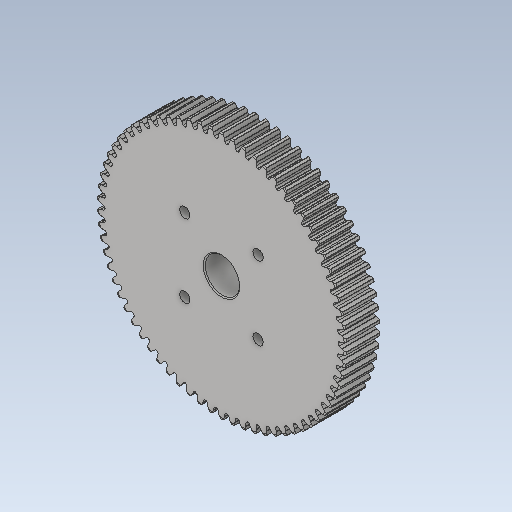
# Autodesk Inventor part: GEABP1.0-70-10-B-10-KFC30-K3_b
Saved by Autodesk Inventor 2020.2 (Build 242310000, 310)
## iProperties
Created: 2022-11-02
Part Number: GEABP1.0-70-10-B-10-KFC30-K3_b
Material: Generic
Catalog Web Link: www.cadenas.de
Description: GEABM, GEABMS, GEABMT, GEABP, GEABPS, GEABPT, GEABA, GEABAS, GEABAT_body-Plastic Spur Gears - Pressure Angle 20 Degrees, Module 0.5/0.8/1.0/1.5/2.0/2.5/3.0
Vendor: MISUMI
Document SubType Name: Modeling
Designer: psAdmin
Manufacturer: MISUMI
Mass: 48.5724 g
Surface Area: 144.734 cm^2
Volume: 48.5724 cm^3
Density: 1 g/cm^3
Appearance: PSOLRGB-175-175-175
Category: PARTsolutions
Company: MISUMI
PSOL_IDENT_0: {$CADENAS_DATA/23d-libs/misumi/metric/54_spur_gears/geabms20/geabms20.prj},408 {VTYP=3D},{NB=GEABP1.
PSOL_IDENT_1: 0-70-10-B-10-KFC30-K3_b},{LINA=GEABP1.0-70-10-B-10-KFC30-K3},{NN=GEABM, GEABMS, GEABMT, GEABP, GEABP
PSOL_IDENT_2: S, GEABPT, GEABA, GEABAS, GEABAT_body},{DATE=17.10.2022 23:48:33},{GEOMDATE=14.09.2022 05:11:00},{VE
PSOL_IDENT_3: RSION=},{LINEID=30},{WBVAR=MATSG,MATCR,NT,B,TS,PS,ALT1,ALT2,TPC,ALT11,ALT10,BS,ALT3,Z,J,ALT4,Q,R,S,T
PSOL_IDENT_4: ,ALT5,LFC,LTC,MALT5,ALT6,KFC,KTC,K},{WBNUMERIC=NT,B,BS,Z,J,Q,R,S,T,LFC,LTC,KFC,KTC,K}  {NB=GEABP1.0-
PSOL_IDENT_5: 70-10-B-10-KFC30-K3_b},{LINA=GEABP1.0-70-10-B-10-KFC30-K3},{KT=DUMMY},{PN=GEABP1.0-70-10-B-10-KFC30-
PSOL_IDENT_6: K3},{TYPE=GEABP},{MATSG=PW},{MATSGALG='MCN','MC Nylon','PW','Polyacetal White','PB','Polyacetal Blue'
PSOL_IDENT_7: },{MATCR=},{MATCRALG='','-','S45C','1045 Carbon Steel','SUS304','304 Stainless Steel'},{MOD=1.0},{MO
PSOL_IDENT_8: D1=1.0},{NT=70},{NTALG=15,16,18,20,22,24,25,26,28,30,32,35,36,40,45,48,50,55,60,70,75,80,90,100,120}
PSOL_IDENT_9: ,{B=10},{BALG=10,15},{TS=B},{TSALG='A','A','B','B'},{TSPN=-B},{PS=10},{PSALG='10','10','11','11','12'
PSOL_IDENT_10: ,'12','13','13','14','14','15','15','16','16','17','17','18','18','19','19','20','20','21','21','22'
PSOL_IDENT_11: ,'22','23','23','24','24','25','25','26','26','27','27','28','28'},{PSCRL='10','10','11','11','12','
PSOL_IDENT_12: 12','13','13','14','14','15','15','16','16','17','17','18','18','19','19','20','20','21','21','22','
PSOL_IDENT_13: 22','23','23','24','24','25','25','26','26','27','27','28','28'},{PSCRW='10','10','12','12','15','15'
PSOL_IDENT_14: ,'20','20'},{DD=70.0},{DD05=35},{DD08=56},{DD10=70},{DD15=105},{DD20=0},{DD25=0},{DD30=0},{D=72.0},{
PSOL_IDENT_15: D05=36},{D08=57.6},{D10=72},{D15=108},{D20=0},{D25=0},{D30=0},{G=67.50},{G05=33.75},{G08=54},{G10=67
PSOL_IDENT_16: .5},{G15=101.25},{G20=0},{G25=0},{G30=0},{H=40.0},{L=20},{LL1=10},{LL2=4.0},{M=M4},{M3D=4},{P=10.00}
PSOL_IDENT_17: ,{DD1=0},{CIFR=15},{CIFM=4},{CIFK=0},{CIFTAP=1},{ALT1=},{ALT1ALG='','w/o Set Screw','KC90','with KC9
PSOL_IDENT_18: 0 (Set Screw)','KC120','with KC120 (Set Screw)'},{ALT1PN=},{ALT2=},{ALT2ALG='','w/o TPC (Tapped Hole
PSOL_IDENT_19: Dimension)','TPC','with TPC (Tapped Hole Dimension)'},{TPC=N/A},{TPCALG='N/A'},{ALT2PN=},{KC=0},{AL
PSOL_IDENT_20: T11=},{ALT11ALG='', 'w/o GBA (Gear bottom adjustment of phase focus)', 'GBA', 'with GBA (Gear bottom
PSOL_IDENT_21: adjustment of phase focus)' },{ALT11PN=},{DEG=0},{ALT10=},{ALT10ALG= '','w/o BS (Boss Cut)','BS','w
PSOL_IDENT_22: ith BS (Boss Cut)' },{ALT10PN=},{BS=0.0},{BSALG=0},{BSMIN=7},{BSMINALG=7.000},{BSMAX=10},{LL13D=10},
PSOL_IDENT_23: {LL23D=16},{LBS=20},{ALT3=},{ALT3ALG= '','w/o Stepped Hole','DHL','with DHL (Stepped Hole)','DHR','w
PSOL_IDENT_24: ith DHR (Stepped Hole)' },{ALT3PN=},{ZJPN=},{ALT31=1},{ALT32=1},{Z=0},{ZALG=0},{ZMINL=12},{ZMAXL=63}
PSOL_IDENT_25: ,{ZMINR=12},{ZMAXR=36},{ZPN=},{J=0.0},{JALG=0},{JMIN=2},{JMAX=0},{JPN=},{ALT4=},{ALT4ALG= '','w/o WD
PSOL_IDENT_26: H (Both Ends Stepped Hole)','WDH','with WDH (Both Ends Stepped Hole)' },{ALT4PN=},{QRSTPN=},{LB=20.0
PSOL_IDENT_27: 00},{Q=0},{QALG=0},{QMIN=12},{QMAX=36},{QPN=},{R=0},{RALG=0},{RMIN=12},{RMAX=36},{RPN=},{S=0},{SALG=
PSOL_IDENT_28: 0},{SMIN=3},{SMAX=14},{SPN=},{T=0},{TALG=0},{TMIN=3},{TMAX=0},{TPN=},{ALT5=},{ALT5ALG= '','Not appli
PSOL_IDENT_29: cable' },{LFC=0},{LFCALG=0},{LTC=0},{LTCALG=0},{LPCDMIN=18},{LPCDMAX=60},{LCMAX=63},{MALT5=N/A},{MAL
PSOL_IDENT_30: T5ALG= 'N/A' },{LCMAX2=60},{C=0.0},{ALT5PN=},{ALT6=KFC},{ALT6ALG= '','w/o Side Through Hole','KFC','
PSOL_IDENT_31: with KFC (Side Through Hole)','KTC','with KTC (Side Through Hole)' },{ALT6PN=-KFC},{KFTCPN=30-K3},{K
PSOL_IDENT_32: FC=30},{KFCALG=[17:33/1],[47:60/1]},{KFCPN=30},{KTC=0},{KTCALG=[0]},{KTCPN=},{KPCDMIN1=17},{KPCDMAX1=
PSOL_IDENT_33: 33},{KPCDMIN2=47},{KPCDMAX2=60},{K=3.0},{KALG=[3:6/0.5]},{KPCD=30},{KPN=-K3},{SCREW=4},{SCREWL=3},{A
PSOL_IDENT_34: G=0},{PCD=30},{SHN=4},{SHDEG1=45},{SHDEG2=90},{PZQRDD2=10},{D1=1.285714},{D2=2.571429},{D3=20},{D4=0
PSOL_IDENT_35: .1},{D5=11.666667},{D6=10.769231},{D7=0.85},{D8=0.5},{D9=0.82917},{S1=15},{S2=0.5},{KR=15}
NB: GEABP1.0-70-10-B-10-KFC30-K3_b
NN: GEABM, GEABMS, GEABMT, GEABP, GEABPS, GEABPT, GEABA, GEABAS, GEABAT_body
NT: 70
NBSYN: $PN._b
LINA: GEABP1.0-70-10-B-10-KFC30-K3
CATALOG: Misumi
PN: GEABP1.0-70-10-B-10-KFC30-K3
MATSG: Polyacetal White
MATCR: -
MOD: 1.0
B: 10
TS: B
PS: 10
DD: 70
D: 72
G: 67.5
H: 40
L: 20
LL1: 10
LL2: 4
M: M4
DD1: 0
ALT1: w/o Set Screw
ALT2: w/o TPC (Tapped Hole Dimension)
TPC: N/A
ALT11: w/o GBA (Gear bottom adjustment of phase focus)
ALT10: w/o BS (Boss Cut)
BS: 0
ALT3: w/o Stepped Hole
Z: 0
J: 0
ALT4: w/o WDH (Both Ends Stepped Hole)
Q: 0
R: 0
S: 0
T: 0
ALT5: Not applicable
LFC: 0
LTC: 0
MALT5: N/A
C: 0
ALT6: with KFC (Side Through Hole)
KFC: 30
KTC: 0
K: 3
SUPPLIER: MISUMI
ARTICLENO: GEABP1.0-70-10-B-10-KFC30-K3_b
BOMINFO: GEABP1.0-70-10-B-10-KFC30-K3
CREATOR: CADENAS GmbH
Title: GEABP1.0-70-10-B-10-KFC30-K3
Author: Cadenas PARTsolutions
Comments: Plastic Spur Gears - Pressure Angle 20 Degrees, Module 0.5/0.8/1.0/1.5/2.0/2.5/3.0
Autodesk Inventor part; units mm, degrees
(part 1 of 2)
sketch "Sketch_2" plane through (0, 0, 0) normal (1, 0, 0) x (0, 1, 0)
  line L0 (0, -500) -> (0, 500)
  line L1 (0, 0) -> (35.5, 0)
  line L2 (35.5, 0) -> (38, -0.6699)
  line L3 (38, -0.6699) -> (38, -9.3301)
  line L4 (38, -9.3301) -> (35.5, -10)
  line L5 (35.5, -10) -> (20, -10)
  line L6 (20, -10) -> (20, -19.7)
  line L7 (20, -19.7) -> (19.7, -20)
  line L8 (19.7, -20) -> (0, -20)
  line L9 (0, -20) -> (0, 0)
  constraints: 20 end point
revolve "Revolution1" add sketch "Sketch_2" angle 360 about axis through (0, 0, -500) along (0, 0, -1)
sketch "_____12" plane through (0, 0, 0) normal (0, 0, 1) x (1, 0, 0)
  circle A0 centre (0, 0) radius 144
  arc A1 (-35.9769, 1.2884) -> (-35.9213, 1.1952) centre (-35.877, 1.2849) ccw
  arc A2 (-35.9213, 1.1952) -> (-34.9912, 0.7853) centre (-30.756, 11.6561) ccw
  arc A3 (-34.9912, 0.7853) -> (-34.8755, 0.7497) centre (-34.6902, 1.5579) ccw
  arc A4 (-34.1021, 0.5416) -> (-34.8755, 0.7497) centre (-37.2859, -9.7463) ccw
  arc A5 (-33.7499, 0.063) -> (-34.1021, 0.5416) centre (-34.2499, 0.0639) ccw
  arc A6 (-33.7499, 0.063) -> (-33.7499, -0.063) centre (0, 0) ccw
  arc A7 (-34.1021, -0.5416) -> (-33.7499, -0.063) centre (-34.2499, -0.0639) ccw
  arc A8 (-34.8755, -0.7497) -> (-34.1021, -0.5416) centre (-37.2859, 9.7463) ccw
  arc A9 (-34.8755, -0.7497) -> (-34.9912, -0.7853) centre (-34.6902, -1.5579) ccw
  arc A10 (-34.9912, -0.7853) -> (-35.9213, -1.1952) centre (-30.756, -11.6561) ccw
  arc A11 (-35.9213, -1.1952) -> (-35.9769, -1.2884) centre (-35.877, -1.2849) ccw
  arc A12 (-35.9769, -1.2884) -> (-35.9476, -1.9417) centre (0, 0) ccw
  arc A13 (-35.9476, -1.9417) -> (-35.8838, -2.0296) centre (-35.8477, -1.9363) ccw
  arc A14 (-35.8838, -2.0296) -> (-34.9207, -2.3544) centre (-31.677, 8.8523) ccw
  arc A15 (-34.9207, -2.3544) -> (-34.8023, -2.3795) centre (-34.6902, -1.5579) ccw
  arc A16 (-34.0134, -2.5175) -> (-34.8023, -2.3795) centre (-36.2622, -13.0493) ccw
  arc A17 (-33.6197, -2.9626) -> (-34.0134, -2.5175) centre (-34.1178, -3.0065) ccw
  arc A18 (-33.6197, -2.9626) -> (-33.6084, -3.0881) centre (0, 0) ccw
  arc A19 (-33.9163, -3.5963) -> (-33.6084, -3.0881) centre (-34.1063, -3.1338) ccw
  arc A20 (-34.6679, -3.8729) -> (-33.9163, -3.5963) centre (-38.0095, 6.3647) ccw
  arc A21 (-34.6679, -3.8729) -> (-34.7799, -3.9188) centre (-34.4109, -4.6613) ccw
  arc A22 (-34.7799, -3.9188) -> (-35.6695, -4.4104) centre (-29.5873, -14.3661) ccw
  arc A23 (-35.6695, -4.4104) -> (-35.7166, -4.5082) centre (-35.6174, -4.4957) ccw
  arc A24 (-35.7166, -4.5082) -> (-35.6288, -5.1562) centre (0, 0) ccw
  arc A25 (-35.6288, -5.1562) -> (-35.5574, -5.238) centre (-35.5299, -5.1419) ccw
  arc A26 (-35.5574, -5.238) -> (-34.5691, -5.4752) centre (-32.343, 5.9771) ccw
  arc A27 (-34.5691, -5.4752) -> (-34.4489, -5.4896) centre (-34.4109, -4.6613) ccw
  arc A28 (-33.6508, -5.5563) -> (-34.4489, -5.4896) centre (-34.9465, -16.2473) ccw
  arc A29 (-33.2188, -5.9643) -> (-33.6508, -5.5563) centre (-33.7109, -6.0527) ccw
  arc A30 (-33.2188, -5.9643) -> (-33.1963, -6.0883) centre (0, 0) ccw
  arc A31 (-33.4574, -6.622) -> (-33.1963, -6.0883) centre (-33.6881, -6.1785) ccw
  arc A32 (-34.1812, -6.965) -> (-33.4574, -6.622) centre (-38.427, 2.932) ccw
  arc A33 (-34.1812, -6.965) -> (-34.2886, -7.0206) centre (-33.8545, -7.7271) ccw
  arc A34 (-34.2886, -7.0206) -> (-35.1306, -7.59) centre (-28.1804, -16.9605) ccw
  arc A35 (-35.1306, -7.59) -> (-35.1687, -7.6917) centre (-35.071, -7.6703) ccw
  arc A36 (-35.1687, -7.6917) -> (-35.0232, -8.3292) centre (0, 0) ccw
  arc A37 (-35.0232, -8.3292) -> (-34.9447, -8.4042) centre (-34.9259, -8.306) ccw
  arc A38 (-34.9447, -8.4042) -> (-33.9391, -8.5519) centre (-32.7486, 3.0538) ccw
  arc A39 (-33.9391, -8.5519) -> (-33.8182, -8.5554) centre (-33.8545, -7.7271) ccw
  arc A40 (-33.0173, -8.5504) -> (-33.8182, -8.5554) centre (-33.3494, -19.3145) ccw
  arc A41 (-32.5504, -8.918) -> (-33.0173, -8.5504) centre (-33.0327, -9.0501) ccw
  arc A42 (-32.5504, -8.918) -> (-32.5169, -9.0395) centre (0, 0) ccw
  arc A43 (-32.7291, -9.5945) -> (-32.5169, -9.0395) centre (-32.9987, -9.1734) ccw
  arc A44 (-33.4192, -10.0009) -> (-32.7291, -9.5945) centre (-38.5351, -0.5244) ccw
  arc A45 (-33.4192, -10.0009) -> (-33.5213, -10.066) centre (-33.0256, -10.7307) ccw
  arc A46 (-33.5213, -10.066) -> (-34.3088, -10.7085) centre (-26.5467, -19.4183) ccw
  arc A47 (-34.3088, -10.7085) -> (-34.3377, -10.8132) centre (-34.2423, -10.7832) ccw
  arc A48 (-34.3377, -10.8132) -> (-34.1356, -11.4351) centre (0, 0) ccw
  arc A49 (-34.1356, -11.4351) -> (-34.0507, -11.5028) centre (-34.0408, -11.4033) ccw
  arc A50 (-34.0507, -11.5028) -> (-33.0359, -11.5598) centre (-32.8905, 0.106) ccw
  arc A51 (-33.0359, -11.5598) -> (-32.9151, -11.5524) centre (-33.0256, -10.7307) ccw
  arc A52 (-32.1179, -11.4756) -> (-32.9151, -11.5524) centre (-31.4838, -22.2261) ccw
  arc A53 (-31.62, -11.7999) -> (-32.1179, -11.4756) centre (-32.0885, -11.9747) ccw
  arc A54 (-31.62, -11.7999) -> (-31.5757, -11.9179) centre (0, 0) ccw
  arc A55 (-31.7373, -12.4897) -> (-31.5757, -11.9179) centre (-32.0435, -12.0944) ccw
  arc A56 (-32.3882, -12.9563) -> (-31.7373, -12.4897) centre (-38.333, -3.9765) ccw
  arc A57 (-32.3882, -12.9563) -> (-32.484, -13.0303) centre (-31.9307, -13.6479) ccw
  arc A58 (-32.484, -13.0303) -> (-33.2108, -13.7408) centre (-24.6991, -21.7197) ccw
  arc A59 (-33.2108, -13.7408) -> (-33.2301, -13.8477) centre (-33.1378, -13.8092) ccw
  arc A60 (-33.2301, -13.8477) -> (-32.9731, -14.449) centre (0, 0) ccw
  arc A61 (-32.9731, -14.449) -> (-32.8825, -14.5088) centre (-32.8815, -14.4088) ccw
  arc A62 (-32.8825, -14.5088) -> (-31.8667, -14.4745) centre (-32.7676, -2.8427) ccw
  arc A63 (-31.8667, -14.4745) -> (-31.747, -14.4564) centre (-31.9307, -13.6479) ccw
  arc A64 (-30.9599, -14.3084) -> (-31.747, -14.4564) centre (-29.3647, -24.9588) ccw
  arc A65 (-30.435, -14.5868) -> (-30.9599, -14.3084) centre (-30.8859, -14.8029) ccw
  arc A66 (-30.435, -14.5868) -> (-30.3803, -14.7003) centre (0, 0) ccw
  arc A67 (-30.49, -15.2843) -> (-30.3803, -14.7003) centre (-30.8304, -14.9181) ccw
  arc A68 (-31.0964, -15.8074) -> (-30.49, -15.2843) centre (-37.8222, -7.3967) ccw
  arc A69 (-31.0964, -15.8074) -> (-31.1852, -15.8897) centre (-30.5788, -16.4552) ccw
  arc A70 (-31.1852, -15.8897) -> (-31.8454, -16.6625) centre (-22.6528, -23.8463) ccw
  arc A71 (-31.8454, -16.6625) -> (-31.8551, -16.7707) centre (-31.7666, -16.7241) ccw
  arc A72 (-31.8551, -16.7707) -> (-31.5452, -17.3465) centre (0, 0) ccw
  arc A73 (-31.5452, -17.3465) -> (-31.4496, -17.398) centre (-31.4576, -17.2983) ccw
  arc A74 (-31.4496, -17.398) -> (-30.4409, -17.2728) centre (-32.3808, -5.7685) ccw
  arc A75 (-30.4409, -17.2728) -> (-30.3234, -17.244) centre (-30.5788, -16.4552) ccw
  arc A76 (-29.5527, -17.026) -> (-30.3234, -17.244) centre (-27.0092, -27.4906) ccw
  arc A77 (-29.0049, -17.2562) -> (-29.5527, -17.026) centre (-29.4346, -17.5119) ccw
  arc A78 (-29.0049, -17.2562) -> (-28.9403, -17.3644) centre (0, 0) ccw
  arc A79 (-28.9971, -17.9559) -> (-28.9403, -17.3644) centre (-29.369, -17.6216) ccw
  arc A80 (-29.5543, -18.5312) -> (-28.9971, -17.9559) centre (-37.0069, -10.7572) ccw
  arc A81 (-29.5543, -18.5312) -> (-29.6353, -18.6211) centre (-28.9807, -19.13) ccw
  arc A82 (-29.6353, -18.6211) -> (-30.2236, -19.45) centre (-20.424, -25.7809) ccw
  arc A83 (-30.2236, -19.45) -> (-30.2235, -19.5586) centre (-30.1396, -19.5043) ccw
  arc A84 (-30.2235, -19.5586) -> (-29.8633, -20.1043) centre (0, 0) ccw
  arc A85 (-29.8633, -20.1043) -> (-29.7634, -20.1471) centre (-29.7803, -20.0485) ccw
  arc A86 (-29.7634, -20.1471) -> (-28.7701, -19.932) centre (-31.7334, -8.6479) ccw
  arc A87 (-28.7701, -19.932) -> (-28.6556, -19.8928) centre (-28.9807, -19.13) ccw
  arc A88 (-27.9075, -19.6066) -> (-28.6556, -19.8928) centre (-24.4362, -29.801) ccw
  arc A89 (-27.3413, -19.7868) -> (-27.9075, -19.6066) centre (-27.7464, -20.0799) ccw
  arc A90 (-27.3413, -19.7868) -> (-27.2672, -19.8887) centre (0, 0) ccw
  arc A91 (-27.2709, -20.4829) -> (-27.2672, -19.8887) centre (-27.6712, -20.1833) ccw
  arc A92 (-27.7742, -21.1059) -> (-27.2709, -20.4829) centre (-35.8937, -14.0312) ccw
  arc A93 (-27.7742, -21.1059) -> (-27.8469, -21.2027) centre (-27.1492, -21.6508) ccw
  arc A94 (-27.8469, -21.2027) -> (-28.3584, -22.0809) centre (-18.0308, -27.5079) ccw
  arc A95 (-28.3584, -22.0809) -> (-28.3486, -22.1891) centre (-28.2699, -22.1275) ccw
  arc A96 (-28.3486, -22.1891) -> (-27.9409, -22.7003) centre (0, 0) ccw
  arc A97 (-27.9409, -22.7003) -> (-27.8377, -22.7339) centre (-27.8633, -22.6373) ccw
  arc A98 (-27.8377, -22.7339) -> (-26.8676, -22.4306) centre (-30.8305, -11.4577) ccw
  arc A99 (-26.8676, -22.4306) -> (-26.757, -22.3813) centre (-27.1492, -21.6508) ccw
  arc A100 (-26.0377, -22.0293) -> (-26.757, -22.3813) centre (-21.6665, -31.8715) ccw
  arc A101 (-25.4576, -22.158) -> (-26.0377, -22.0293) centre (-25.8347, -22.4862) ccw
  arc A102 (-25.4576, -22.158) -> (-25.3747, -22.2528) centre (0, 0) ccw
  arc A103 (-25.325, -22.845) -> (-25.3747, -22.2528) centre (-25.7506, -22.5825) ccw
  arc A104 (-25.7705, -23.5106) -> (-25.325, -22.845) centre (-34.4914, -17.1922) ccw
  arc A105 (-25.7705, -23.5106) -> (-25.8342, -23.6135) centre (-25.0992, -23.9973) ccw
  arc A106 (-25.8342, -23.6135) -> (-26.2649, -24.5341) centre (-15.4924, -29.0134) ccw
  arc A107 (-26.2649, -24.5341) -> (-26.2455, -24.6409) centre (-26.1726, -24.5725) ccw
  arc A108 (-26.2455, -24.6409) -> (-25.7936, -25.1135) centre (0, 0) ccw
  arc A109 (-25.7936, -25.1135) -> (-25.6877, -25.1378) centre (-25.722, -25.0438) ccw
  arc A110 (-25.6877, -25.1378) -> (-24.7487, -24.7487) centre (-29.6793, -14.1751) ccw
  arc A111 (-24.7487, -24.7487) -> (-24.6431, -24.6897) centre (-25.0992, -23.9973) ccw
  arc A112 (-23.9582, -24.2746) -> (-24.6431, -24.6897) centre (-18.7224, -33.6854) ccw
  arc A113 (-23.3689, -24.3508) -> (-23.9582, -24.2746) centre (-23.7151, -24.7115) ccw
  arc A114 (-23.3689, -24.3508) -> (-23.2778, -24.4378) centre (0, 0) ccw
  arc A115 (-23.1753, -25.0231) -> (-23.2778, -24.4378) centre (-23.6226, -24.7999) ccw
  arc A116 (-23.5592, -25.726) -> (-23.1753, -25.0231) centre (-32.8115, -20.2148) ccw
  arc A117 (-23.5592, -25.726) -> (-23.6135, -25.8342) centre (-22.847, -26.1505) ccw
  arc A118 (-23.6135, -25.8342) -> (-23.96, -26.7897) centre (-12.8293, -30.2854) ccw
  arc A119 (-23.96, -26.7897) -> (-23.931, -26.8943) centre (-23.8646, -26.8196) ccw
  arc A120 (-23.931, -26.8943) -> (-23.4386, -27.3246) centre (0, 0) ccw
  arc A121 (-23.4386, -27.3246) -> (-23.331, -27.3392) centre (-23.3735, -27.2487) ccw
  arc A122 (-23.331, -27.3392) -> (-22.4306, -26.8676) centre (-28.2892, -16.7785) ccw
  arc A123 (-22.4306, -26.8676) -> (-22.3307, -26.7993) centre (-22.847, -26.1505) ccw
  arc A124 (-21.6857, -26.3244) -> (-22.3307, -26.7993) centre (-15.6275, -35.228) ccw
  arc A125 (-21.092, -26.3475) -> (-21.6857, -26.3244) centre (-21.4045, -26.7378) ccw
  arc A126 (-21.092, -26.3475) -> (-20.9935, -26.426) centre (0, 0) ccw
  arc A127 (-20.8389, -26.9998) -> (-20.9935, -26.426) centre (-21.3045, -26.8175) ccw
  arc A128 (-21.1584, -27.7342) -> (-20.8389, -26.9998) centre (-30.8673, -23.0746) ccw
  arc A129 (-21.1584, -27.7342) -> (-21.2027, -27.8469) centre (-20.4109, -28.0932) ccw
  arc A130 (-21.2027, -27.8469) -> (-21.4621, -28.8296) centre (-10.0629, -31.3135) ccw
  arc A131 (-21.4621, -28.8296) -> (-21.4239, -28.9312) centre (-21.3644, -28.8509) ccw
  arc A132 (-21.4239, -28.9312) -> (-20.8949, -29.3156) centre (0, 0) ccw
  arc A133 (-20.8949, -29.3156) -> (-20.7864, -29.3205) centre (-20.8368, -29.2342) ccw
  arc A134 (-20.7864, -29.3205) -> (-19.932, -28.7701) centre (-26.6713, -19.2468) ccw
  arc A135 (-19.932, -28.7701) -> (-19.8385, -28.6931) centre (-20.4109, -28.0932) ccw
  arc A136 (-19.2387, -28.1624) -> (-19.8385, -28.6931) centre (-12.4067, -36.487) ccw
  arc A137 (-18.6453, -28.1321) -> (-19.2387, -28.1624) centre (-18.9215, -28.5489) ccw
  arc A138 (-18.6453, -28.1321) -> (-18.5402, -28.2015) centre (0, 0) ccw
  arc A139 (-18.3348, -28.7591) -> (-18.5402, -28.2015) centre (-18.8148, -28.6193) ccw
  arc A140 (-18.5871, -29.5192) -> (-18.3348, -28.7591) centre (-28.6747, -25.7486) ccw
  arc A141 (-18.5871, -29.5192) -> (-18.6211, -29.6353) centre (-17.8105, -29.8098) ccw
  arc A142 (-18.6211, -29.6353) -> (-18.7914, -30.6374) centre (-7.2155, -32.0894) ccw
  arc A143 (-18.7914, -30.6374) -> (-18.7443, -30.7352) centre (-18.6922, -30.6498) ccw
  arc A144 (-18.7443, -30.7352) -> (-18.1829, -31.0706) centre (0, 0) ccw
  arc A145 (-18.1829, -31.0706) -> (-18.0745, -31.0657) centre (-18.1324, -30.9843) ccw
  arc A146 (-18.0745, -31.0657) -> (-17.2728, -30.4409) centre (-24.8386, -21.5601) ccw
  arc A147 (-17.2728, -30.4409) -> (-17.1866, -30.3559) centre (-17.8105, -29.8098) ccw
  arc A148 (-16.6368, -29.7735) -> (-17.1866, -30.3559) centre (-9.0861, -37.4523) ccw
  arc A149 (-16.0485, -29.6902) -> (-16.6368, -29.7735) centre (-16.2863, -30.1301) ccw
  arc A150 (-16.0485, -29.6902) -> (-15.9376, -29.7499) centre (0, 0) ccw
  arc A151 (-15.683, -30.2868) -> (-15.9376, -29.7499) centre (-16.1737, -30.1906) ccw
  arc A152 (-15.8662, -31.0665) -> (-15.683, -30.2868) centre (-26.2511, -28.2154) ccw
  arc A153 (-15.8662, -31.0665) -> (-15.8897, -31.1852) centre (-15.0667, -31.2863) ccw
  arc A154 (-15.8897, -31.1852) -> (-15.9695, -32.1985) centre (-4.31, -32.607) ccw
  arc A155 (-15.9695, -32.1985) -> (-15.9137, -32.2917) centre (-15.8695, -32.202) ccw
  arc A156 (-15.9137, -32.2917) -> (-15.3246, -32.5754) centre (0, 0) ccw
  arc A157 (-15.3246, -32.5754) -> (-15.217, -32.5609) centre (-15.282, -32.4849) ccw
  arc A158 (-15.217, -32.5609) -> (-14.4745, -31.8667) centre (-22.806, -23.6998) ccw
  arc A159 (-14.4745, -31.8667) -> (-14.3964, -31.7743) centre (-15.0667, -31.2863) ccw
  arc A160 (-13.901, -31.145) -> (-14.3964, -31.7743) centre (-5.6923, -38.116) ccw
  arc A161 (-13.3225, -31.0092) -> (-13.901, -31.145) centre (-13.5199, -31.4686) ccw
  arc A162 (-13.3225, -31.0092) -> (-13.2066, -31.0588) centre (0, 0) ccw
  arc A163 (-12.905, -31.5707) -> (-13.2066, -31.0588) centre (-13.4023, -31.5189) ccw
  arc A164 (-13.0175, -32.3637) -> (-12.905, -31.5707) centre (-23.6163, -30.4549) ccw
  arc A165 (-13.0175, -32.3637) -> (-13.0303, -32.484) centre (-12.2015, -32.5109) ccw
  arc A166 (-13.0303, -32.484) -> (-13.0189, -33.5004) centre (-1.3697, -32.8621) ccw
  arc A167 (-13.0189, -33.5004) -> (-12.9551, -33.5882) centre (-12.9191, -33.4949) ccw
  arc A168 (-12.9551, -33.5882) -> (-12.3429, -33.8179) centre (0, 0) ccw
  arc A169 (-12.3429, -33.8179) -> (-12.237, -33.7938) centre (-12.3086, -33.724) ccw
  arc A170 (-12.237, -33.7938) -> (-11.5598, -33.0359) centre (-20.5897, -25.6487) ccw
  arc A171 (-11.5598, -33.0359) -> (-11.4902, -32.9369) centre (-12.2015, -32.5109) ccw
  arc A172 (-11.0532, -32.2657) -> (-11.4902, -32.9369) centre (-2.2527, -38.4728) ccw
  arc A173 (-10.4892, -32.0786) -> (-11.0532, -32.2657) centre (-10.6446, -32.5539) ccw
  arc A174 (-10.4892, -32.0786) -> (-10.3694, -32.1176) centre (0, 0) ccw
  arc A175 (-10.0231, -32.6004) -> (-10.3694, -32.1176) centre (-10.523, -32.5934) ccw
  arc A176 (-10.0641, -33.4003) -> (-10.0231, -32.6004) centre (-20.7912, -32.4493) ccw
  arc A177 (-10.0641, -33.4003) -> (-10.066, -33.5213) centre (-9.2382, -33.4738) ccw
  arc A178 (-10.066, -33.5213) -> (-9.9636, -34.5325) centre (1.5815, -32.8526) ccw
  arc A179 (-9.9636, -34.5325) -> (-9.8921, -34.6143) centre (-9.8646, -34.5181) ccw
  arc A180 (-9.8921, -34.6143) -> (-9.2618, -34.7882) centre (0, 0) ccw
  arc A181 (-9.2618, -34.7882) -> (-9.1585, -34.7547) centre (-9.236, -34.6916) ccw
  arc A182 (-9.1585, -34.7547) -> (-8.5519, -33.9391) centre (-18.2077, -27.3911) ccw
  arc A183 (-8.5519, -33.9391) -> (-8.4915, -33.8343) centre (-9.2382, -33.4738) ccw
  arc A184 (-8.1164, -33.1266) -> (-8.4915, -33.8343) centre (1.205, -38.5198) ccw
  arc A185 (-7.5715, -32.8897) -> (-8.1164, -33.1266) centre (-7.6837, -33.377) ccw
  arc A186 (-7.5715, -32.8897) -> (-7.4487, -32.9178) centre (0, 0) ccw
  arc A187 (-7.0604, -33.3676) -> (-7.4487, -32.9178) centre (-7.559, -33.4054) ccw
  arc A188 (-7.0296, -34.1679) -> (-7.0604, -33.3676) centre (-17.7988, -34.1823) ccw
  arc A189 (-7.0296, -34.1679) -> (-7.0206, -34.2886) centre (-6.2004, -34.1671) ccw
  arc A190 (-7.0206, -34.2886) -> (-6.828, -35.2866) centre (4.52, -32.5786) ccw
  arc A191 (-6.828, -35.2866) -> (-6.7495, -35.3616) centre (-6.7307, -35.2634) ccw
  arc A192 (-6.7495, -35.3616) -> (-6.1061, -35.4784) centre (0, 0) ccw
  arc A193 (-6.1061, -35.4784) -> (-6.0062, -35.4357) centre (-6.0891, -35.3798) ccw
  arc A194 (-6.0062, -35.4357) -> (-5.4752, -34.5691) centre (-15.6791, -28.913) ccw
  arc A195 (-5.4752, -34.5691) -> (-5.4244, -34.4592) centre (-6.2004, -34.1671) ccw
  arc A196 (-5.1143, -33.7208) -> (-5.4244, -34.4592) centre (4.6531, -38.2567) ccw
  arc A197 (-4.5928, -33.436) -> (-5.1143, -33.7208) centre (-4.6608, -33.9314) ccw
  arc A198 (-4.5928, -33.436) -> (-4.4679, -33.453) centre (0, 0) ccw
  arc A199 (-4.041, -33.8662) -> (-4.4679, -33.453) centre (-4.5341, -33.9486) ccw
  arc A200 (-3.9385, -34.6605) -> (-4.041, -33.8662) centre (-14.6631, -35.6402) ccw
  arc A201 (-3.9385, -34.6605) -> (-3.9188, -34.7799) centre (-3.1127, -34.5854) ccw
  arc A202 (-3.9188, -34.7799) -> (-3.6374, -35.7566) centre (7.4222, -32.0423) ccw
  arc A203 (-3.6374, -35.7566) -> (-3.5525, -35.8243) centre (-3.5426, -35.7248) ccw
  arc A204 (-3.5525, -35.8243) -> (-2.9013, -35.8829) centre (0, 0) ccw
  arc A205 (-2.9013, -35.8829) -> (-2.8056, -35.8315) centre (-2.8932, -35.7832) ccw
  arc A206 (-2.8056, -35.8315) -> (-2.3544, -34.9207) centre (-13.0242, -30.202) ccw
  arc A207 (-2.3544, -34.9207) -> (-2.3137, -34.8068) centre (-3.1127, -34.5854) ccw
  arc A208 (-2.071, -34.0435) -> (-2.3137, -34.8068) centre (8.0636, -37.6856) ccw
  arc A209 (-1.5771, -33.7131) -> (-2.071, -34.0435) centre (-1.6005, -34.2126) ccw
  arc A210 (-1.5771, -33.7131) -> (-1.4513, -33.7188) centre (0, 0) ccw
  arc A211 (-0.989, -34.0921) -> (-1.4513, -33.7188) centre (-1.4728, -34.2183) ccw
  arc A212 (-0.8157, -34.874) -> (-0.989, -34.0921) centre (-11.4093, -36.8111) ccw
  arc A213 (-0.8157, -34.874) -> (-0.7853, -34.9912) centre (0, -34.7251) ccw
  arc A214 (-0.7853, -34.9912) -> (-0.4176, -35.9387) centre (10.2645, -31.2479) ccw
  arc A215 (-0.4176, -35.9387) -> (-0.3269, -35.9985) centre (-0.326, -35.8985) ccw
  arc A216 (-0.3269, -35.9985) -> (0.3269, -35.9985) centre (0, 0) ccw
  arc A217 (0.3269, -35.9985) -> (0.4176, -35.9387) centre (0.326, -35.8985) ccw
  arc A218 (0.4176, -35.9387) -> (0.7853, -34.9912) centre (-10.2645, -31.2479) ccw
  arc A219 (0.7853, -34.9912) -> (0.8157, -34.874) centre (0, -34.7251) ccw
  arc A220 (0.989, -34.0921) -> (0.8157, -34.874) centre (11.4093, -36.8111) ccw
  arc A221 (1.4513, -33.7188) -> (0.989, -34.0921) centre (1.4728, -34.2183) ccw
  arc A222 (1.4513, -33.7188) -> (1.5771, -33.7131) centre (0, 0) ccw
  arc A223 (2.071, -34.0435) -> (1.5771, -33.7131) centre (1.6005, -34.2126) ccw
  arc A224 (2.3137, -34.8068) -> (2.071, -34.0435) centre (-8.0636, -37.6856) ccw
  arc A225 (2.3137, -34.8068) -> (2.3544, -34.9207) centre (3.1127, -34.5854) ccw
  arc A226 (2.3544, -34.9207) -> (2.8056, -35.8315) centre (13.0242, -30.202) ccw
  arc A227 (2.8056, -35.8315) -> (2.9013, -35.8829) centre (2.8932, -35.7832) ccw
  arc A228 (2.9013, -35.8829) -> (3.5525, -35.8243) centre (0, 0) ccw
  arc A229 (3.5525, -35.8243) -> (3.6374, -35.7566) centre (3.5426, -35.7248) ccw
  arc A230 (3.6374, -35.7566) -> (3.9188, -34.7799) centre (-7.4222, -32.0423) ccw
  arc A231 (3.9188, -34.7799) -> (3.9385, -34.6605) centre (3.1127, -34.5854) ccw
  arc A232 (4.041, -33.8662) -> (3.9385, -34.6605) centre (14.6631, -35.6402) ccw
  arc A233 (4.4679, -33.453) -> (4.041, -33.8662) centre (4.5341, -33.9486) ccw
  arc A234 (4.4679, -33.453) -> (4.5928, -33.436) centre (0, 0) ccw
  arc A235 (5.1143, -33.7208) -> (4.5928, -33.436) centre (4.6608, -33.9314) ccw
  arc A236 (5.4244, -34.4592) -> (5.1143, -33.7208) centre (-4.6531, -38.2567) ccw
  arc A237 (5.4244, -34.4592) -> (5.4752, -34.5691) centre (6.2004, -34.1671) ccw
  arc A238 (5.4752, -34.5691) -> (6.0062, -35.4357) centre (15.6791, -28.913) ccw
  arc A239 (6.0062, -35.4357) -> (6.1061, -35.4784) centre (6.0891, -35.3798) ccw
  arc A240 (6.1061, -35.4784) -> (6.7495, -35.3616) centre (0, 0) ccw
  arc A241 (6.7495, -35.3616) -> (6.828, -35.2866) centre (6.7307, -35.2634) ccw
  arc A242 (6.828, -35.2866) -> (7.0206, -34.2886) centre (-4.52, -32.5786) ccw
  arc A243 (7.0206, -34.2886) -> (7.0296, -34.1679) centre (6.2004, -34.1671) ccw
  arc A244 (7.0604, -33.3676) -> (7.0296, -34.1679) centre (17.7988, -34.1823) ccw
  arc A245 (7.4487, -32.9178) -> (7.0604, -33.3676) centre (7.559, -33.4054) ccw
  arc A246 (7.4487, -32.9178) -> (7.5715, -32.8897) centre (0, 0) ccw
  arc A247 (8.1164, -33.1266) -> (7.5715, -32.8897) centre (7.6837, -33.377) ccw
  arc A248 (8.4915, -33.8343) -> (8.1164, -33.1266) centre (-1.205, -38.5198) ccw
  arc A249 (8.4915, -33.8343) -> (8.5519, -33.9391) centre (9.2382, -33.4738) ccw
  arc A250 (8.5519, -33.9391) -> (9.1585, -34.7547) centre (18.2077, -27.3911) ccw
  arc A251 (9.1585, -34.7547) -> (9.2618, -34.7882) centre (9.236, -34.6916) ccw
  arc A252 (9.2618, -34.7882) -> (9.8921, -34.6143) centre (0, 0) ccw
  arc A253 (9.8921, -34.6143) -> (9.9636, -34.5325) centre (9.8646, -34.5181) ccw
  arc A254 (9.9636, -34.5325) -> (10.066, -33.5213) centre (-1.5815, -32.8526) ccw
  arc A255 (10.066, -33.5213) -> (10.0641, -33.4003) centre (9.2382, -33.4738) ccw
  arc A256 (10.0231, -32.6004) -> (10.0641, -33.4003) centre (20.7912, -32.4493) ccw
  arc A257 (10.3694, -32.1176) -> (10.0231, -32.6004) centre (10.523, -32.5934) ccw
  arc A258 (10.3694, -32.1176) -> (10.4892, -32.0786) centre (0, 0) ccw
  arc A259 (11.0532, -32.2657) -> (10.4892, -32.0786) centre (10.6446, -32.5539) ccw
  arc A260 (11.4902, -32.9369) -> (11.0532, -32.2657) centre (2.2527, -38.4728) ccw
  arc A261 (11.4902, -32.9369) -> (11.5598, -33.0359) centre (12.2015, -32.5109) ccw
  arc A262 (11.5598, -33.0359) -> (12.237, -33.7938) centre (20.5897, -25.6487) ccw
  arc A263 (12.237, -33.7938) -> (12.3429, -33.8179) centre (12.3086, -33.724) ccw
  arc A264 (12.3429, -33.8179) -> (12.9551, -33.5882) centre (0, 0) ccw
  arc A265 (12.9551, -33.5882) -> (13.0189, -33.5004) centre (12.9191, -33.4949) ccw
  arc A266 (13.0189, -33.5004) -> (13.0303, -32.484) centre (1.3697, -32.8621) ccw
  arc A267 (13.0303, -32.484) -> (13.0175, -32.3637) centre (12.2015, -32.5109) ccw
  arc A268 (12.905, -31.5707) -> (13.0175, -32.3637) centre (23.6163, -30.4549) ccw
  arc A269 (13.2066, -31.0588) -> (12.905, -31.5707) centre (13.4023, -31.5189) ccw
  arc A270 (13.2066, -31.0588) -> (13.3225, -31.0092) centre (0, 0) ccw
  arc A271 (13.901, -31.145) -> (13.3225, -31.0092) centre (13.5199, -31.4686) ccw
  arc A272 (14.3964, -31.7743) -> (13.901, -31.145) centre (5.6923, -38.116) ccw
  arc A273 (14.3964, -31.7743) -> (14.4745, -31.8667) centre (15.0667, -31.2863) ccw
  arc A274 (14.4745, -31.8667) -> (15.217, -32.5609) centre (22.806, -23.6998) ccw
  arc A275 (15.217, -32.5609) -> (15.3246, -32.5754) centre (15.282, -32.4849) ccw
  arc A276 (15.3246, -32.5754) -> (15.9137, -32.2917) centre (0, 0) ccw
  arc A277 (15.9137, -32.2917) -> (15.9695, -32.1985) centre (15.8695, -32.202) ccw
  arc A278 (15.9695, -32.1985) -> (15.8897, -31.1852) centre (4.31, -32.607) ccw
  arc A279 (15.8897, -31.1852) -> (15.8662, -31.0665) centre (15.0667, -31.2863) ccw
  arc A280 (15.683, -30.2868) -> (15.8662, -31.0665) centre (26.2511, -28.2154) ccw
  arc A281 (15.9376, -29.7499) -> (15.683, -30.2868) centre (16.1737, -30.1906) ccw
  arc A282 (15.9376, -29.7499) -> (16.0485, -29.6902) centre (0, 0) ccw
  arc A283 (16.6368, -29.7735) -> (16.0485, -29.6902) centre (16.2863, -30.1301) ccw
  arc A284 (17.1866, -30.3559) -> (16.6368, -29.7735) centre (9.0861, -37.4523) ccw
  arc A285 (17.1866, -30.3559) -> (17.2728, -30.4409) centre (17.8105, -29.8098) ccw
  arc A286 (17.2728, -30.4409) -> (18.0745, -31.0657) centre (24.8386, -21.5601) ccw
  arc A287 (18.0745, -31.0657) -> (18.1829, -31.0706) centre (18.1324, -30.9843) ccw
  arc A288 (18.1829, -31.0706) -> (18.7443, -30.7352) centre (0, 0) ccw
  arc A289 (18.7443, -30.7352) -> (18.7914, -30.6374) centre (18.6922, -30.6498) ccw
  arc A290 (18.7914, -30.6374) -> (18.6211, -29.6353) centre (7.2155, -32.0894) ccw
  arc A291 (18.6211, -29.6353) -> (18.5871, -29.5192) centre (17.8105, -29.8098) ccw
  arc A292 (18.3348, -28.7591) -> (18.5871, -29.5192) centre (28.6747, -25.7486) ccw
  arc A293 (18.5402, -28.2015) -> (18.3348, -28.7591) centre (18.8148, -28.6193) ccw
  arc A294 (18.5402, -28.2015) -> (18.6453, -28.1321) centre (0, 0) ccw
  arc A295 (19.2387, -28.1624) -> (18.6453, -28.1321) centre (18.9215, -28.5489) ccw
  arc A296 (19.8385, -28.6931) -> (19.2387, -28.1624) centre (12.4067, -36.487) ccw
  arc A297 (19.8385, -28.6931) -> (19.932, -28.7701) centre (20.4109, -28.0932) ccw
  arc A298 (19.932, -28.7701) -> (20.7864, -29.3205) centre (26.6713, -19.2468) ccw
  arc A299 (20.7864, -29.3205) -> (20.8949, -29.3156) centre (20.8368, -29.2342) ccw
  arc A300 (20.8949, -29.3156) -> (21.4239, -28.9312) centre (0, 0) ccw
  arc A301 (21.4239, -28.9312) -> (21.4621, -28.8296) centre (21.3644, -28.8509) ccw
  arc A302 (21.4621, -28.8296) -> (21.2027, -27.8469) centre (10.0629, -31.3135) ccw
  arc A303 (21.2027, -27.8469) -> (21.1584, -27.7342) centre (20.4109, -28.0932) ccw
  arc A304 (20.8389, -26.9998) -> (21.1584, -27.7342) centre (30.8673, -23.0746) ccw
  arc A305 (20.9935, -26.426) -> (20.8389, -26.9998) centre (21.3045, -26.8175) ccw
  arc A306 (20.9935, -26.426) -> (21.092, -26.3475) centre (0, 0) ccw
  arc A307 (21.6857, -26.3244) -> (21.092, -26.3475) centre (21.4045, -26.7378) ccw
  arc A308 (22.3307, -26.7993) -> (21.6857, -26.3244) centre (15.6275, -35.228) ccw
  arc A309 (22.3307, -26.7993) -> (22.4306, -26.8676) centre (22.847, -26.1505) ccw
  arc A310 (22.4306, -26.8676) -> (23.331, -27.3392) centre (28.2892, -16.7785) ccw
  arc A311 (23.331, -27.3392) -> (23.4386, -27.3246) centre (23.3735, -27.2487) ccw
  arc A312 (23.4386, -27.3246) -> (23.931, -26.8943) centre (0, 0) ccw
  arc A313 (23.931, -26.8943) -> (23.96, -26.7897) centre (23.8646, -26.8196) ccw
  arc A314 (23.96, -26.7897) -> (23.6135, -25.8342) centre (12.8293, -30.2854) ccw
  arc A315 (23.6135, -25.8342) -> (23.5592, -25.726) centre (22.847, -26.1505) ccw
  arc A316 (23.1753, -25.0231) -> (23.5592, -25.726) centre (32.8115, -20.2148) ccw
  arc A317 (23.2778, -24.4378) -> (23.1753, -25.0231) centre (23.6226, -24.7999) ccw
  arc A318 (23.2778, -24.4378) -> (23.3689, -24.3508) centre (0, 0) ccw
  arc A319 (23.9582, -24.2746) -> (23.3689, -24.3508) centre (23.7151, -24.7115) ccw
  arc A320 (24.6431, -24.6897) -> (23.9582, -24.2746) centre (18.7224, -33.6854) ccw
  arc A321 (24.6431, -24.6897) -> (24.7487, -24.7487) centre (25.0992, -23.9973) ccw
  arc A322 (24.7487, -24.7487) -> (25.6877, -25.1378) centre (29.6793, -14.1751) ccw
  arc A323 (25.6877, -25.1378) -> (25.7936, -25.1135) centre (25.722, -25.0438) ccw
  arc A324 (25.7936, -25.1135) -> (26.2455, -24.6409) centre (0, 0) ccw
  arc A325 (26.2455, -24.6409) -> (26.2649, -24.5341) centre (26.1726, -24.5725) ccw
  arc A326 (26.2649, -24.5341) -> (25.8342, -23.6135) centre (15.4924, -29.0134) ccw
  arc A327 (25.8342, -23.6135) -> (25.7705, -23.5106) centre (25.0992, -23.9973) ccw
  arc A328 (25.325, -22.845) -> (25.7705, -23.5106) centre (34.4914, -17.1922) ccw
  arc A329 (25.3747, -22.2528) -> (25.325, -22.845) centre (25.7506, -22.5825) ccw
  arc A330 (25.3747, -22.2528) -> (25.4576, -22.158) centre (0, 0) ccw
  arc A331 (26.0377, -22.0293) -> (25.4576, -22.158) centre (25.8347, -22.4862) ccw
  arc A332 (26.757, -22.3813) -> (26.0377, -22.0293) centre (21.6665, -31.8715) ccw
  arc A333 (26.757, -22.3813) -> (26.8676, -22.4306) centre (27.1492, -21.6508) ccw
  arc A334 (26.8676, -22.4306) -> (27.8377, -22.7339) centre (30.8305, -11.4577) ccw
  arc A335 (27.8377, -22.7339) -> (27.9409, -22.7003) centre (27.8633, -22.6373) ccw
  arc A336 (27.9409, -22.7003) -> (28.3486, -22.1891) centre (0, 0) ccw
  arc A337 (28.3486, -22.1891) -> (28.3584, -22.0809) centre (28.2699, -22.1275) ccw
  arc A338 (28.3584, -22.0809) -> (27.8469, -21.2027) centre (18.0308, -27.5079) ccw
  arc A339 (27.8469, -21.2027) -> (27.7742, -21.1059) centre (27.1492, -21.6508) ccw
  arc A340 (27.2709, -20.4829) -> (27.7742, -21.1059) centre (35.8937, -14.0312) ccw
  arc A341 (27.2672, -19.8887) -> (27.2709, -20.4829) centre (27.6712, -20.1833) ccw
  arc A342 (27.2672, -19.8887) -> (27.3413, -19.7868) centre (0, 0) ccw
  arc A343 (27.9075, -19.6066) -> (27.3413, -19.7868) centre (27.7464, -20.0799) ccw
  arc A344 (28.6556, -19.8928) -> (27.9075, -19.6066) centre (24.4362, -29.801) ccw
  arc A345 (28.6556, -19.8928) -> (28.7701, -19.932) centre (28.9807, -19.13) ccw
  arc A346 (28.7701, -19.932) -> (29.7634, -20.1471) centre (31.7334, -8.6479) ccw
  arc A347 (29.7634, -20.1471) -> (29.8633, -20.1043) centre (29.7803, -20.0485) ccw
  arc A348 (29.8633, -20.1043) -> (30.2235, -19.5586) centre (0, 0) ccw
  arc A349 (30.2235, -19.5586) -> (30.2236, -19.45) centre (30.1396, -19.5043) ccw
  arc A350 (30.2236, -19.45) -> (29.6353, -18.6211) centre (20.424, -25.7809) ccw
  arc A351 (29.6353, -18.6211) -> (29.5543, -18.5312) centre (28.9807, -19.13) ccw
  arc A352 (28.9971, -17.9559) -> (29.5543, -18.5312) centre (37.0069, -10.7572) ccw
  arc A353 (28.9403, -17.3644) -> (28.9971, -17.9559) centre (29.369, -17.6216) ccw
  arc A354 (28.9403, -17.3644) -> (29.0049, -17.2562) centre (0, 0) ccw
  arc A355 (29.5527, -17.026) -> (29.0049, -17.2562) centre (29.4346, -17.5119) ccw
  arc A356 (30.3234, -17.244) -> (29.5527, -17.026) centre (27.0092, -27.4906) ccw
  arc A357 (30.3234, -17.244) -> (30.4409, -17.2728) centre (30.5788, -16.4552) ccw
  arc A358 (30.4409, -17.2728) -> (31.4496, -17.398) centre (32.3808, -5.7685) ccw
  arc A359 (31.4496, -17.398) -> (31.5452, -17.3465) centre (31.4576, -17.2983) ccw
  arc A360 (31.5452, -17.3465) -> (31.8551, -16.7707) centre (0, 0) ccw
  arc A361 (31.8551, -16.7707) -> (31.8454, -16.6625) centre (31.7666, -16.7241) ccw
  arc A362 (31.8454, -16.6625) -> (31.1852, -15.8897) centre (22.6528, -23.8463) ccw
  arc A363 (31.1852, -15.8897) -> (31.0964, -15.8074) centre (30.5788, -16.4552) ccw
  arc A364 (30.49, -15.2843) -> (31.0964, -15.8074) centre (37.8222, -7.3967) ccw
  arc A365 (30.3803, -14.7003) -> (30.49, -15.2843) centre (30.8304, -14.9181) ccw
  arc A366 (30.3803, -14.7003) -> (30.435, -14.5868) centre (0, 0) ccw
  arc A367 (30.9599, -14.3084) -> (30.435, -14.5868) centre (30.8859, -14.8029) ccw
  arc A368 (31.747, -14.4564) -> (30.9599, -14.3084) centre (29.3647, -24.9588) ccw
  arc A369 (31.747, -14.4564) -> (31.8667, -14.4745) centre (31.9307, -13.6479) ccw
  arc A370 (31.8667, -14.4745) -> (32.8825, -14.5088) centre (32.7676, -2.8427) ccw
  arc A371 (32.8825, -14.5088) -> (32.9731, -14.449) centre (32.8815, -14.4088) ccw
  arc A372 (32.9731, -14.449) -> (33.2301, -13.8477) centre (0, 0) ccw
  arc A373 (33.2301, -13.8477) -> (33.2108, -13.7408) centre (33.1378, -13.8092) ccw
  arc A374 (33.2108, -13.7408) -> (32.484, -13.0303) centre (24.6991, -21.7197) ccw
  arc A375 (32.484, -13.0303) -> (32.3882, -12.9563) centre (31.9307, -13.6479) ccw
  arc A376 (31.7373, -12.4897) -> (32.3882, -12.9563) centre (38.333, -3.9765) ccw
  arc A377 (31.5757, -11.9179) -> (31.7373, -12.4897) centre (32.0435, -12.0944) ccw
  arc A378 (31.5757, -11.9179) -> (31.62, -11.7999) centre (0, 0) ccw
  arc A379 (32.1179, -11.4756) -> (31.62, -11.7999) centre (32.0885, -11.9747) ccw
  arc A380 (32.9151, -11.5524) -> (32.1179, -11.4756) centre (31.4838, -22.2261) ccw
  arc A381 (32.9151, -11.5524) -> (33.0359, -11.5598) centre (33.0256, -10.7307) ccw
  arc A382 (33.0359, -11.5598) -> (34.0507, -11.5028) centre (32.8905, 0.106) ccw
  arc A383 (34.0507, -11.5028) -> (34.1356, -11.4351) centre (34.0408, -11.4033) ccw
  arc A384 (34.1356, -11.4351) -> (34.3377, -10.8132) centre (0, 0) ccw
  arc A385 (34.3377, -10.8132) -> (34.3088, -10.7085) centre (34.2423, -10.7832) ccw
  arc A386 (34.3088, -10.7085) -> (33.5213, -10.066) centre (26.5467, -19.4183) ccw
  arc A387 (33.5213, -10.066) -> (33.4192, -10.0009) centre (33.0256, -10.7307) ccw
  arc A388 (32.7291, -9.5945) -> (33.4192, -10.0009) centre (38.5351, -0.5244) ccw
  arc A389 (32.5169, -9.0395) -> (32.7291, -9.5945) centre (32.9987, -9.1734) ccw
  arc A390 (32.5169, -9.0395) -> (32.5504, -8.918) centre (0, 0) ccw
  arc A391 (33.0173, -8.5504) -> (32.5504, -8.918) centre (33.0327, -9.0501) ccw
  arc A392 (33.8182, -8.5554) -> (33.0173, -8.5504) centre (33.3494, -19.3145) ccw
  arc A393 (33.8182, -8.5554) -> (33.9391, -8.5519) centre (33.8545, -7.7271) ccw
  arc A394 (33.9391, -8.5519) -> (34.9447, -8.4042) centre (32.7486, 3.0538) ccw
  arc A395 (34.9447, -8.4042) -> (35.0232, -8.3292) centre (34.9259, -8.306) ccw
  arc A396 (35.0232, -8.3292) -> (35.1687, -7.6917) centre (0, 0) ccw
  arc A397 (35.1687, -7.6917) -> (35.1306, -7.59) centre (35.071, -7.6703) ccw
  arc A398 (35.1306, -7.59) -> (34.2886, -7.0206) centre (28.1804, -16.9605) ccw
  arc A399 (34.2886, -7.0206) -> (34.1812, -6.965) centre (33.8545, -7.7271) ccw
  arc A400 (33.4574, -6.622) -> (34.1812, -6.965) centre (38.427, 2.932) ccw
  arc A401 (33.1963, -6.0883) -> (33.4574, -6.622) centre (33.6881, -6.1785) ccw
  arc A402 (33.1963, -6.0883) -> (33.2188, -5.9643) centre (0, 0) ccw
  arc A403 (33.6508, -5.5563) -> (33.2188, -5.9643) centre (33.7109, -6.0527) ccw
  arc A404 (34.4489, -5.4896) -> (33.6508, -5.5563) centre (34.9465, -16.2473) ccw
  arc A405 (34.4489, -5.4896) -> (34.5691, -5.4752) centre (34.4109, -4.6613) ccw
  arc A406 (34.5691, -5.4752) -> (35.5574, -5.238) centre (32.343, 5.9771) ccw
  arc A407 (35.5574, -5.238) -> (35.6288, -5.1562) centre (35.5299, -5.1419) ccw
  arc A408 (35.6288, -5.1562) -> (35.7166, -4.5082) centre (0, 0) ccw
  arc A409 (35.7166, -4.5082) -> (35.6695, -4.4104) centre (35.6174, -4.4957) ccw
  arc A410 (35.6695, -4.4104) -> (34.7799, -3.9188) centre (29.5873, -14.3661) ccw
  arc A411 (34.7799, -3.9188) -> (34.6679, -3.8729) centre (34.4109, -4.6613) ccw
  arc A412 (33.9163, -3.5963) -> (34.6679, -3.8729) centre (38.0095, 6.3647) ccw
  arc A413 (33.6084, -3.0881) -> (33.9163, -3.5963) centre (34.1063, -3.1338) ccw
  arc A414 (33.6084, -3.0881) -> (33.6197, -2.9626) centre (0, 0) ccw
  arc A415 (34.0134, -2.5175) -> (33.6197, -2.9626) centre (34.1178, -3.0065) ccw
  arc A416 (34.8023, -2.3795) -> (34.0134, -2.5175) centre (36.2622, -13.0493) ccw
  arc A417 (34.8023, -2.3795) -> (34.9207, -2.3544) centre (34.6902, -1.5579) ccw
  arc A418 (34.9207, -2.3544) -> (35.8838, -2.0296) centre (31.677, 8.8523) ccw
  arc A419 (35.8838, -2.0296) -> (35.9476, -1.9417) centre (35.8477, -1.9363) ccw
  arc A420 (35.9476, -1.9417) -> (35.9769, -1.2884) centre (0, 0) ccw
  arc A421 (35.9769, -1.2884) -> (35.9213, -1.1952) centre (35.877, -1.2849) ccw
  arc A422 (35.9213, -1.1952) -> (34.9912, -0.7853) centre (30.756, -11.6561) ccw
  arc A423 (34.9912, -0.7853) -> (34.8755, -0.7497) centre (34.6902, -1.5579) ccw
  arc A424 (34.1021, -0.5416) -> (34.8755, -0.7497) centre (37.2859, 9.7463) ccw
  arc A425 (33.7499, -0.063) -> (34.1021, -0.5416) centre (34.2499, -0.0639) ccw
  arc A426 (33.7499, -0.063) -> (33.7499, 0.063) centre (0, 0) ccw
  arc A427 (34.1021, 0.5416) -> (33.7499, 0.063) centre (34.2499, 0.0639) ccw
  arc A428 (34.8755, 0.7497) -> (34.1021, 0.5416) centre (37.2859, -9.7463) ccw
  arc A429 (34.8755, 0.7497) -> (34.9912, 0.7853) centre (34.6902, 1.5579) ccw
  arc A430 (34.9912, 0.7853) -> (35.9213, 1.1952) centre (30.756, 11.6561) ccw
  arc A431 (35.9213, 1.1952) -> (35.9769, 1.2884) centre (35.877, 1.2849) ccw
  arc A432 (35.9769, 1.2884) -> (35.9476, 1.9417) centre (0, 0) ccw
  arc A433 (35.9476, 1.9417) -> (35.8838, 2.0296) centre (35.8477, 1.9363) ccw
  arc A434 (35.8838, 2.0296) -> (34.9207, 2.3544) centre (31.677, -8.8523) ccw
  arc A435 (34.9207, 2.3544) -> (34.8023, 2.3795) centre (34.6902, 1.5579) ccw
  arc A436 (34.0134, 2.5175) -> (34.8023, 2.3795) centre (36.2622, 13.0493) ccw
  arc A437 (33.6197, 2.9626) -> (34.0134, 2.5175) centre (34.1178, 3.0065) ccw
  arc A438 (33.6197, 2.9626) -> (33.6084, 3.0881) centre (0, 0) ccw
  arc A439 (33.9163, 3.5963) -> (33.6084, 3.0881) centre (34.1063, 3.1338) ccw
  arc A440 (34.6679, 3.8729) -> (33.9163, 3.5963) centre (38.0095, -6.3647) ccw
  arc A441 (34.6679, 3.8729) -> (34.7799, 3.9188) centre (34.4109, 4.6613) ccw
  arc A442 (34.7799, 3.9188) -> (35.6695, 4.4104) centre (29.5873, 14.3661) ccw
  arc A443 (35.6695, 4.4104) -> (35.7166, 4.5082) centre (35.6174, 4.4957) ccw
  arc A444 (35.7166, 4.5082) -> (35.6288, 5.1562) centre (0, 0) ccw
  arc A445 (35.6288, 5.1562) -> (35.5574, 5.238) centre (35.5299, 5.1419) ccw
  arc A446 (35.5574, 5.238) -> (34.5691, 5.4752) centre (32.343, -5.9771) ccw
  arc A447 (34.5691, 5.4752) -> (34.4489, 5.4896) centre (34.4109, 4.6613) ccw
  arc A448 (33.6508, 5.5563) -> (34.4489, 5.4896) centre (34.9465, 16.2473) ccw
  arc A449 (33.2188, 5.9643) -> (33.6508, 5.5563) centre (33.7109, 6.0527) ccw
  arc A450 (33.2188, 5.9643) -> (33.1963, 6.0883) centre (0, 0) ccw
  arc A451 (33.4574, 6.622) -> (33.1963, 6.0883) centre (33.6881, 6.1785) ccw
  arc A452 (34.1812, 6.965) -> (33.4574, 6.622) centre (38.427, -2.932) ccw
  arc A453 (34.1812, 6.965) -> (34.2886, 7.0206) centre (33.8545, 7.7271) ccw
  arc A454 (34.2886, 7.0206) -> (35.1306, 7.59) centre (28.1804, 16.9605) ccw
  arc A455 (35.1306, 7.59) -> (35.1687, 7.6917) centre (35.071, 7.6703) ccw
  arc A456 (35.1687, 7.6917) -> (35.0232, 8.3292) centre (0, 0) ccw
  arc A457 (35.0232, 8.3292) -> (34.9447, 8.4042) centre (34.9259, 8.306) ccw
  arc A458 (34.9447, 8.4042) -> (33.9391, 8.5519) centre (32.7486, -3.0538) ccw
  arc A459 (33.9391, 8.5519) -> (33.8182, 8.5554) centre (33.8545, 7.7271) ccw
  arc A460 (33.0173, 8.5504) -> (33.8182, 8.5554) centre (33.3494, 19.3145) ccw
  arc A461 (32.5504, 8.918) -> (33.0173, 8.5504) centre (33.0327, 9.0501) ccw
  arc A462 (32.5504, 8.918) -> (32.5169, 9.0395) centre (0, 0) ccw
  arc A463 (32.7291, 9.5945) -> (32.5169, 9.0395) centre (32.9987, 9.1734) ccw
  arc A464 (33.4192, 10.0009) -> (32.7291, 9.5945) centre (38.5351, 0.5244) ccw
  arc A465 (33.4192, 10.0009) -> (33.5213, 10.066) centre (33.0256, 10.7307) ccw
  arc A466 (33.5213, 10.066) -> (34.3088, 10.7085) centre (26.5467, 19.4183) ccw
  arc A467 (34.3088, 10.7085) -> (34.3377, 10.8132) centre (34.2423, 10.7832) ccw
  arc A468 (34.3377, 10.8132) -> (34.1356, 11.4351) centre (0, 0) ccw
  arc A469 (34.1356, 11.4351) -> (34.0507, 11.5028) centre (34.0408, 11.4033) ccw
  arc A470 (34.0507, 11.5028) -> (33.0359, 11.5598) centre (32.8905, -0.106) ccw
  arc A471 (33.0359, 11.5598) -> (32.9151, 11.5524) centre (33.0256, 10.7307) ccw
  arc A472 (32.1179, 11.4756) -> (32.9151, 11.5524) centre (31.4838, 22.2261) ccw
  arc A473 (31.62, 11.7999) -> (32.1179, 11.4756) centre (32.0885, 11.9747) ccw
  arc A474 (31.62, 11.7999) -> (31.5757, 11.9179) centre (0, 0) ccw
  arc A475 (31.7373, 12.4897) -> (31.5757, 11.9179) centre (32.0435, 12.0944) ccw
  arc A476 (32.3882, 12.9563) -> (31.7373, 12.4897) centre (38.333, 3.9765) ccw
  arc A477 (32.3882, 12.9563) -> (32.484, 13.0303) centre (31.9307, 13.6479) ccw
  arc A478 (32.484, 13.0303) -> (33.2108, 13.7408) centre (24.6991, 21.7197) ccw
  arc A479 (33.2108, 13.7408) -> (33.2301, 13.8477) centre (33.1378, 13.8092) ccw
  arc A480 (33.2301, 13.8477) -> (32.9731, 14.449) centre (0, 0) ccw
  arc A481 (32.9731, 14.449) -> (32.8825, 14.5088) centre (32.8815, 14.4088) ccw
  arc A482 (32.8825, 14.5088) -> (31.8667, 14.4745) centre (32.7676, 2.8427) ccw
  arc A483 (31.8667, 14.4745) -> (31.747, 14.4564) centre (31.9307, 13.6479) ccw
  arc A484 (30.9599, 14.3084) -> (31.747, 14.4564) centre (29.3647, 24.9588) ccw
  arc A485 (30.435, 14.5868) -> (30.9599, 14.3084) centre (30.8859, 14.8029) ccw
  arc A486 (30.435, 14.5868) -> (30.3803, 14.7003) centre (0, 0) ccw
  arc A487 (30.49, 15.2843) -> (30.3803, 14.7003) centre (30.8304, 14.9181) ccw
  arc A488 (31.0964, 15.8074) -> (30.49, 15.2843) centre (37.8222, 7.3967) ccw
  arc A489 (31.0964, 15.8074) -> (31.1852, 15.8897) centre (30.5788, 16.4552) ccw
  arc A490 (31.1852, 15.8897) -> (31.8454, 16.6625) centre (22.6528, 23.8463) ccw
  arc A491 (31.8454, 16.6625) -> (31.8551, 16.7707) centre (31.7666, 16.7241) ccw
  arc A492 (31.8551, 16.7707) -> (31.5452, 17.3465) centre (0, 0) ccw
  arc A493 (31.5452, 17.3465) -> (31.4496, 17.398) centre (31.4576, 17.2983) ccw
  arc A494 (31.4496, 17.398) -> (30.4409, 17.2728) centre (32.3808, 5.7685) ccw
  arc A495 (30.4409, 17.2728) -> (30.3234, 17.244) centre (30.5788, 16.4552) ccw
  arc A496 (29.5527, 17.026) -> (30.3234, 17.244) centre (27.0092, 27.4906) ccw
  arc A497 (29.0049, 17.2562) -> (29.5527, 17.026) centre (29.4346, 17.5119) ccw
  arc A498 (29.0049, 17.2562) -> (28.9403, 17.3644) centre (0, 0) ccw
  arc A499 (28.9971, 17.9559) -> (28.9403, 17.3644) centre (29.369, 17.6216) ccw
  arc A500 (29.5543, 18.5312) -> (28.9971, 17.9559) centre (37.0069, 10.7572) ccw
  arc A501 (29.5543, 18.5312) -> (29.6353, 18.6211) centre (28.9807, 19.13) ccw
  arc A502 (29.6353, 18.6211) -> (30.2236, 19.45) centre (20.424, 25.7809) ccw
  arc A503 (30.2236, 19.45) -> (30.2235, 19.5586) centre (30.1396, 19.5043) ccw
  arc A504 (30.2235, 19.5586) -> (29.8633, 20.1043) centre (0, 0) ccw
  arc A505 (29.8633, 20.1043) -> (29.7634, 20.1471) centre (29.7803, 20.0485) ccw
  arc A506 (29.7634, 20.1471) -> (28.7701, 19.932) centre (31.7334, 8.6479) ccw
  arc A507 (28.7701, 19.932) -> (28.6556, 19.8928) centre (28.9807, 19.13) ccw
  arc A508 (27.9075, 19.6066) -> (28.6556, 19.8928) centre (24.4362, 29.801) ccw
  arc A509 (27.3413, 19.7868) -> (27.9075, 19.6066) centre (27.7464, 20.0799) ccw
  arc A510 (27.3413, 19.7868) -> (27.2672, 19.8887) centre (0, 0) ccw
  arc A511 (27.2709, 20.4829) -> (27.2672, 19.8887) centre (27.6712, 20.1833) ccw
  arc A512 (27.7742, 21.1059) -> (27.2709, 20.4829) centre (35.8937, 14.0312) ccw
  arc A513 (27.7742, 21.1059) -> (27.8469, 21.2027) centre (27.1492, 21.6508) ccw
  arc A514 (27.8469, 21.2027) -> (28.3584, 22.0809) centre (18.0308, 27.5079) ccw
  arc A515 (28.3584, 22.0809) -> (28.3486, 22.1891) centre (28.2699, 22.1275) ccw
  arc A516 (28.3486, 22.1891) -> (27.9409, 22.7003) centre (0, 0) ccw
  arc A517 (27.9409, 22.7003) -> (27.8377, 22.7339) centre (27.8633, 22.6373) ccw
  arc A518 (27.8377, 22.7339) -> (26.8676, 22.4306) centre (30.8305, 11.4577) ccw
  arc A519 (26.8676, 22.4306) -> (26.757, 22.3813) centre (27.1492, 21.6508) ccw
  arc A520 (26.0377, 22.0293) -> (26.757, 22.3813) centre (21.6665, 31.8715) ccw
  arc A521 (25.4576, 22.158) -> (26.0377, 22.0293) centre (25.8347, 22.4862) ccw
  arc A522 (25.4576, 22.158) -> (25.3747, 22.2528) centre (0, 0) ccw
  arc A523 (25.325, 22.845) -> (25.3747, 22.2528) centre (25.7506, 22.5825) ccw
  arc A524 (25.7705, 23.5106) -> (25.325, 22.845) centre (34.4914, 17.1922) ccw
  arc A525 (25.7705, 23.5106) -> (25.8342, 23.6135) centre (25.0992, 23.9973) ccw
  arc A526 (25.8342, 23.6135) -> (26.2649, 24.5341) centre (15.4924, 29.0134) ccw
  arc A527 (26.2649, 24.5341) -> (26.2455, 24.6409) centre (26.1726, 24.5725) ccw
  arc A528 (26.2455, 24.6409) -> (25.7936, 25.1135) centre (0, 0) ccw
  arc A529 (25.7936, 25.1135) -> (25.6877, 25.1378) centre (25.722, 25.0438) ccw
  arc A530 (25.6877, 25.1378) -> (24.7487, 24.7487) centre (29.6793, 14.1751) ccw
  arc A531 (24.7487, 24.7487) -> (24.6431, 24.6897) centre (25.0992, 23.9973) ccw
  arc A532 (23.9582, 24.2746) -> (24.6431, 24.6897) centre (18.7224, 33.6854) ccw
  arc A533 (23.3689, 24.3508) -> (23.9582, 24.2746) centre (23.7151, 24.7115) ccw